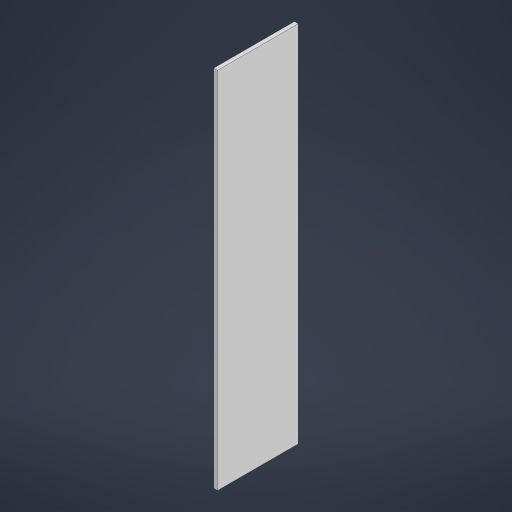
# Autodesk Inventor part: platte_drawing
Saved by Autodesk Inventor 2023 (Build 270158000, 158)
## iProperties
Created: 2022-11-14
Part Number: platte_drawing
Material: Generic
Document SubType Name: Modeling
Designer: bananenbrot
Density: 1 g/cm^3
Appearance: Default
Author: bananenbrot
Autodesk Inventor part; units mm, degrees
ref_plane "YZ Plane" through (0, 0, 0) normal (1, 0, 0) x (0, 1, 0)
ref_plane "XZ Plane" through (0, 0, 0) normal (0, 1, 0) x (-1, 0, 0)
ref_plane "XY Plane" through (0, 0, 0) normal (0, 0, 1) x (1, 0, 0)
sketch "Sketch1" plane through (0, 0, 0) normal (1, 0, 0) x (0, 1, 0)
  line L0 (116.0424, 78.2136) -> (-171.9576, 78.2136)
  line L1 (-171.9576, 78.2136) -> (-171.9576, 14.3136)
  line L2 (-171.9576, 14.3136) -> (116.0424, 14.3136)
  line L3 (116.0424, 14.3136) -> (116.0424, 78.2136)
  point P0 (0, 0)
  dimension "d0" = 63.9
  dimension "d1" = 288
  constraints: 8 end point, 2 parallel, 1 horizontal, 1 perpendicular
  measures "d0" distance of L2.end L0.start
  measures "d1" distance of L0.start L0.end
extrude "Extrusion1" add sketch "Sketch1" along normal blind 3
body "Solid1"
